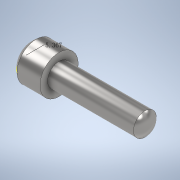
# Autodesk Inventor part: 7-顶轴
Saved by Autodesk Inventor 2022 (Build 260153000, 153)
## iProperties
Created: 2023-01-09
Part Number: 7-顶轴
Material: 不锈钢
Document SubType Name: Modeling
Designer: Lzy18
Density: 8 g/cm^3
Appearance: 半抛光
Author: Lzy18
Autodesk Inventor part; units mm, degrees
ref_plane "YZ Plane" through (0, 0, 0) normal (1, 0, 0) x (0, 1, 0)
ref_plane "XZ Plane" through (0, 0, 0) normal (0, 1, 0) x (-1, 0, 0)
ref_plane "XY Plane" through (0, 0, 0) normal (0, 0, 1) x (1, 0, 0)
sketch "草图1" plane through (0, 0, 0) normal (0, 0, 1) x (1, 0, 0)
  line L0 (0, 0) -> (12, 0)
  line L1 (12, 0) -> (12, -10)
  line L2 (12, -10) -> (0, -10)
  line L3 (0, -10) -> (0, 0)
  line L4 (12, 0) -> (57, 0)
  line L5 (57, 0) -> (57, -6)
  line L6 (57, -6) -> (12, -6)
  line L7 (12, -6) -> (12, 0)
  arc A0 (-5.3668, 0) -> (0, -10) centre (6.6332, 0) ccw
  arc A1 (57, -6) -> (59.7085, 0) centre (51.7085, 0) ccw
  line L8 (-5.3668, 0) -> (0, 0)
  line L9 (57, 0) -> (59.7085, 0)
  dimension "d0" = 12
  dimension "d1" = 10
  dimension "d2" = 45
  dimension "d3" = 6
  dimension "d4" = 24
  dimension "d5" = 16
  constraints: 20 end point, 4 parallel, 4 point on circle, 4 point on line, 2 centre point, 2 collinear, 2 horizontal, 2 perpendicular
  measures "d0" distance of L1.end L2.end
  measures "d1" distance of L0.end L1.end
  measures "d2" distance of L5.end L6.end
  measures "d3" distance of L4.end L5.end
  measures "d4" diameter of A0
  measures "d5" diameter of A1
revolve "旋转1" add sketch "草图1" angle 360 about axis through (12, 0, 0) along (1, 0, 0)
sketch "草图2" plane through (0, 0, 0) normal (0, 1, 0) x (-1, 0, 0)
  line L0 (0, -10) -> (0, 10) projected
  arc A0 (0, -10) -> (0, 10) centre (-6.6332, 0) ccw projected
  point P0 (0, 0)
  point P1 (5.3668, 0)
  dimension "d7" = 5.3667
  constraints: 1 point on circle
  measures "d7" distance from line of point (5.367, 0) L0
